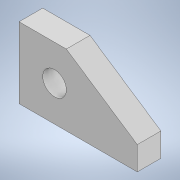
# Autodesk Inventor part: Peça2
Saved by Autodesk Inventor 2021 (Build 250183000, 183)
## iProperties
Created: 2022-02-08
Part Number: Peça2
Material: Genérico
Document SubType Name: Modeling
Designer: aluno
Density: 1 g/cm^3
Appearance: Padrão
Author: aluno
Autodesk Inventor part; units mm, degrees
ref_plane "YZ Plane" through (0, 0, 0) normal (1, 0, 0) x (0, 1, 0)
ref_plane "XZ Plane" through (0, 0, 0) normal (0, 1, 0) x (-1, 0, 0)
ref_plane "XY Plane" through (0, 0, 0) normal (0, 0, 1) x (1, 0, 0)
sketch "Esboço1" plane through (0, 0, 0) normal (0, 0, 1) x (1, 0, 0)
  line L0 (0, 0) -> (50, 0)
  line L1 (50, 0) -> (50, 10)
  line L2 (0, 0) -> (0, 30)
  line L3 (0, 30) -> (20, 30)
  line L4 (20, 30) -> (50, 10)
  dimension "d0" = 50
  dimension "d1" = 10
  dimension "d2" = 30
  dimension "d3" = 20
  constraints: 10 end point, 2 perpendicular, 1 horizontal, 1 vertical
  measures "d0" distance of L0.start L0.end
  measures "d1" distance of L0.end L1.end
  measures "d2" distance of L0.start L2.end
  measures "d3" distance of L2.end L3.end
extrude "Extrusão1" add sketch "Esboço1" along normal blind 10
sketch "Esboço2" plane through (0, 0, 10) normal (0, 0, 1) x (1, 0, 0)
  line L0 (0, 30) -> (0, 0) projected
  line L1 (0, 0) -> (50, 0) projected
  point P0 (15, 15)
  dimension "d6" = 15
  dimension "d14" = 15
  measures "d6" distance from line of L0 point (15, 15)
  measures "d14" distance from line of L1 point (15, 15)
hole "Furo1" at (15, 15, 10) direction (0, 0, -1) diameter 10 end through all
